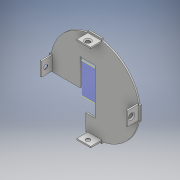
# Autodesk Inventor part: Hull_top
Saved by Autodesk Inventor 2018 (Build 220112000, 112)
## iProperties
Created: 2018-03-12
Part Number: Hull_top
Material: Generic
Document SubType Name: Modeling
Designer: Suchanek
Density: 1 g/cm^3
Appearance: Default
Author: Suchanek
Autodesk Inventor part; units mm, degrees
ref_plane "YZ Plane" through (0, 0, 0) normal (1, 0, 0) x (0, 1, 0)
ref_plane "XZ Plane" through (0, 0, 0) normal (0, 1, 0) x (-1, 0, 0)
ref_plane "XY Plane" through (0, 0, 0) normal (0, 0, 1) x (1, 0, 0)
sketch "Sketch1" plane through (0, 0, 0) normal (0, 1, 0) x (-1, 0, 0)
  arc A0 (31.6389, 4.7938) -> (6.5, -31.3329) centre (0, 0) ccw
  line L0 (-5, 33) -> (5, 33)
  line L1 (5, 33) -> (5, 31.607)
  line L2 (5, -33) -> (-5, -33)
  line L3 (-5, -33) -> (-5, 5)
  line L4 (-5, 33) -> (5, -33) construction
  line L5 (5, 33) -> (-5, -33) construction
  line L6 (-33, 5) -> (-5, 5)
  line L7 (33, 5) -> (33, -5)
  line L8 (33, -5) -> (31.607, -5)
  line L9 (-33, -5) -> (-33, 5)
  line L10 (-33, 5) -> (33, -5) construction
  line L11 (33, 5) -> (-33, -5) construction
  arc A1 (4.7938, -31.6389) -> (6.5, -31.3329) centre (0, 0) ccw
  line L12 (6.5, -31.3329) -> (6.5, -19.2329)
  line L13 (6.5, -19.2329) -> (-0.3, -19.2329)
  line L14 (-0.3, -19.2329) -> (-0.3, -5.7329)
  line L15 (-0.3, 13.7671) -> (5, 13.7671)
  line L16 (10.7, 13.7671) -> (10.7, 5)
  line L17 (10.7, -5.7329) -> (31.4823, -5.7329)
  arc A2 (31.4823, -5.7329) -> (31.607, -5) centre (0, 0) ccw
  arc A3 (31.6389, -4.7938) -> (31.6389, 4.7938) centre (0, 0) ccw
  line L18 (5, -19.2329) -> (5, -33)
  line L19 (5, 13.7671) -> (5, 5)
  line L20 (10.7, 1.6212) -> (10.7, -5.7329)
  line L21 (-0.3, -5) -> (-0.3, 5)
  arc A4 (6.5, -31.3329) -> (10.7, -30.1581) centre (0, 0) ccw
  line L22 (5, -5) -> (0.7576, -5)
  line L23 (5, 5) -> (10.7, 5)
  line L24 (-5, 5) -> (-0.3, 5)
  line L25 (-5, -5) -> (-33, -5)
  line L26 (-5, 5) -> (-5, 33)
  line L27 (5, 5) -> (5, -5)
  line L28 (5, 31.607) -> (5, 13.7671)
  arc A5 (10.7, -30.1581) -> (31.4823, -5.7329) centre (0, 0) ccw
  arc A6 (6.5, -31.3329) -> (31.6389, -4.7938) centre (0, 0) ccw
  line L29 (-0.3, -5.7329) -> (-0.3, -5)
  line L30 (5, -5) -> (5, -5.7329)
  line L31 (10.7, 5) -> (31.607, 5)
  line L32 (10.7, -5) -> (5, -5)
  line L33 (0.7576, 5) -> (5, 5)
  line L34 (-0.3, 5) -> (0.7576, 5)
  line L35 (5, 13.7671) -> (10.7, 13.7671)
  line L36 (-0.3, 5) -> (-0.3, 13.7671)
  line L37 (31.607, 5) -> (33, 5)
  line L38 (10.7, 5) -> (10.7, 1.6212)
  line L39 (31.607, -5) -> (10.7, -5)
  line L40 (0.7576, -5) -> (-5, -5)
  line L41 (5, -5.7329) -> (5, -19.2329)
  dimension "d0" = 64
  dimension "d1" = 10
  dimension "d2" = 66
  dimension "d3" = 66
  dimension "d4" = 10
  dimension "d11" = 12.1
  dimension "d12" = 6.8
  dimension "d13" = 33
  dimension "d14" = 0.3
  dimension "d15" = 11
  dimension "d16" = 19.5
  constraints: 84 end point, 58 parallel, 24 perpendicular, 22 point on circle, 16 point on line, 11 horizontal, 7 centre point, 4 midpoint, 4 vertical, 2 coincident
  measures "d0" diameter of A0
  measures "d1" distance of L2.start L2.end
  measures "d2" distance of L0.end L2.start
  measures "d3" distance of L7.end L9.start
  measures "d4" distance of L7.start L7.end
  measures "d11" distance of L12.start L12.end
  measures "d12" distance of L12.end L13.end
  measures "d13" distance of L13.end L15.start
  measures "d14" distance from line of point (0, 0) L14
  measures "d15" distance of L15.start L16.start
  measures "d16" distance of L16.start L17.start
ref_plane "Work Plane1" through (0, 1, 0) normal (0, 1, 0) x (1, 0, 0)
sketch "Sketch2" plane through (0, 1, 0) normal (0, 1, 0) x (1, 0, 0)
  circle A0 centre (0, 0) radius 33
  dimension "d7" = 66
  constraints: 1 centre point, 1 coincident
  measures "d7" diameter of A0
extrude "Extrusion2" [suppressed]
extrude "Extrusion3" add sketch "Sketch1" along normal blind 1 contours A3 A6 L39 L20 L38 L31 A0 | A0 L37 L7 L8 A6 A3 | L31 L16 L35 L28 A0 | L28 L15 L36 L24 L26 A0 | A0 L26 L0 L1 | A2 L17 L20 L39 | L26 L6 A0 | L6 L3 L25 A0 | A0 L25 L9 L6 | L24 L21 L40 L3 | L25 L3 A0 | L40 L29 L14 L13 L18 A0 L3 | A0 L18 L13 L12 | A0 L18 L2 L3
sketch "Sketch3" plane through (0, 0, 0) normal (0, -1, 0) x (1, 0, 0)
  line L0 (-5, -33) -> (-5, -31.607) projected
  line L1 (-5, -31.607) -> (5, -31.607)
  line L2 (5, -31.607) -> (5, -30.607)
  line L3 (5, -30.607) -> (-5, -30.607)
  line L4 (-5, -30.607) -> (-5, -31.607)
  line L5 (-33, 5) -> (-31.607, 5) projected
  line L6 (-31.607, 5) -> (-30.607, 5)
  line L7 (-30.607, 5) -> (-30.607, -5)
  line L8 (-30.607, -5) -> (-31.607, -5)
  line L9 (-31.607, -5) -> (-31.607, 5)
  line L10 (-5, 31.607) -> (-5, 33) projected
  line L11 (-5, 31.607) -> (5, 31.607)
  line L12 (5, 31.607) -> (5, 30.607)
  line L13 (5, 30.607) -> (-5, 30.607)
  line L14 (-5, 30.607) -> (-5, 31.607)
  line L15 (31.607, 5) -> (30.607, 5)
  line L16 (30.607, 5) -> (30.607, -5)
  line L17 (30.607, -5) -> (31.607, -5)
  line L18 (31.607, -5) -> (31.607, 5)
  line L19 (31.607, 5) -> (33, 5) projected
  dimension "d21" = 10
  dimension "d22" = 1
  dimension "d23" = 1
  dimension "d24" = 10
  dimension "d25" = 10
  dimension "d26" = 1
  dimension "d27" = 1
  dimension "d28" = 10
  constraints: 32 end point, 8 parallel, 4 horizontal, 4 perpendicular, 2 point on line
  measures "d21" distance of L3.end L2.end
  measures "d22" distance of L2.end L1.end
  measures "d23" distance of L7.end L8.end
  measures "d24" distance of L6.end L7.end
  measures "d25" distance of L12.end L13.end
  measures "d26" distance of L11.end L12.end
  measures "d27" distance of L17.end L16.end
  measures "d28" distance of L16.end L15.end
extrude "Extrusion4" add sketch "Sketch3" along normal blind 8
sketch "Sketch4" plane through (31.607, 0, 5) normal (1, 0, 0) x (0, 0, -1)
  circle A0 centre (5, -5) radius 2.295
  line L0 (0, 0) -> (10, 0) projected
  point P0 (5, 0)
  point P1 (5, 0)
  dimension "d31" = 4.59
  dimension "d32" = 5
  constraints: 1 centre point, 1 midpoint, 1 vertical alignment
  measures "d31" diameter of A0
  measures "d32" distance from line of A0.centre L0
hole "Hole1" at (31.607, -5, 0) direction (-1, 0, 0) diameter 3.1 end through all countersink diameter 4.59 countersink angle 90
pattern_circular "Circular Pattern1" count 4 over 360 about axis through (0, 0, 0) along (0, 1, 0) of "Hole1"
body "Solid1"
